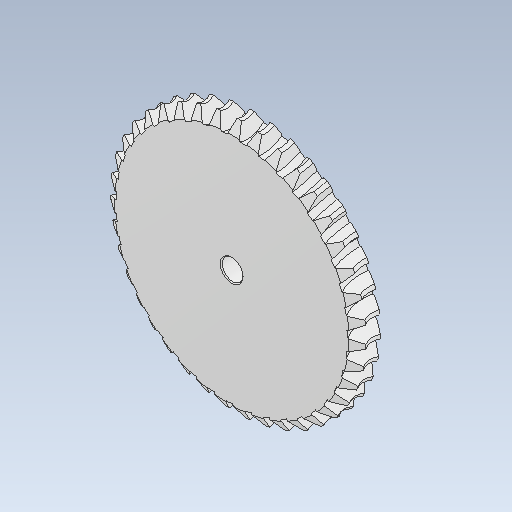
# Autodesk Inventor part: Worm Gear
Saved by Autodesk Inventor 2020 (Build 240168000, 168)
## iProperties
CustomPartVersion: 1
Created: 2020-05-17
Part Number: Worm Gear
Material: Acetal Resin, White
Document SubType Name: Modeling
Designer: Hesekiel
Categories: <?xml version="1.0" encoding="UTF-16"?> <MemberInstance><Categories><FamilyTemplate><FamilyTemplateParameter ValueType="xs:double" Id="1" ObjectReferenceKey="da_z" ObjectType="kUserParameterObject"/><FamilyTemplateParameter ValueType="xs:double" Id="2" ObjectReferenceKey="da_b" ObjectType="kUserParameterObject"/><FamilyTemplateParameter ValueType="xs:double" Id="3" ObjectReferenceKey="da_beta" ObjectType="kUserParameterObject"/><FamilyTemplateParameter ValueType="xs:double" Id="4" ObjectReferenceKey="da_m" ObjectType="kUserParameterObject"/><FamilyTemplateParameter ValueType="xs:double" Id="5" ObjectReferenceKey="da_alpha" ObjectType="kUserParameterObject"/><FamilyTemplateParameter ValueType="xs:double" Id="6" ObjectReferenceKey="da_da" ObjectType="kUserParameterObject"/><FamilyTemplateParameter ValueType="xs:double" Id="7" ObjectReferenceKey="da_aw" ObjectType="kUserParameterObject"/><FamilyTemplateParameter ValueType="xs:double" Id="8" ObjectReferenceKey="da_px" ObjectType="kUserParameterObject"/><FamilyTemplateParameter ValueType="xs:double" Id="9" ObjectReferenceKey="da_d" ObjectType="kUserParameterObject"/><FamilyTemplateParameter ValueType="xs:double" Id="10" ObjectReferenceKey="da_dae" ObjectType="kUserParameterObject"/><FamilyTemplateParameter ValueType="xs:double" Id="11" ObjectReferenceKey="da_fi" ObjectType="kUserParameterObject"/><FamilyTemplateParameter ValueType="xs:string" Id="12" ObjectReferenceKey="EAIAABAAAAAWFwAAAAAAAIAAAAAAAAAA" ObjectType="83910656" SubObjectId="SurfaceGeometry"/></FamilyTemplate><ParamToTemplateMap><ParamToTemplate CategoryParameter="//CategoryParameter[@InternalName='046C89C9-8512-4d59-83FE-43B91F4F132A']" TemplateParameter="1"/><ParamToTemplate CategoryParameter="//CategoryParameter[@InternalName='2552DF32-E462-4b46-AEBF-C6C7768E72AC']" TemplateParameter="2"/><ParamToTemplate CategoryParameter="//CategoryParameter[@InternalName='C9EE641D-15FC-4fae-A226-E94C4372FDD7']" TemplateParameter="3"/><ParamToTemplate><ParamToTemplate CategoryParameter="//CategoryParameter[@InternalName='00B6519A-459B-49c7-AD84-2E56D39A5744']" ConstantValue="-0.427778"/></ParamToTemplate><ParamToTemplate><ParamToTemplate CategoryParameter="//CategoryParameter[@InternalName='04B31F0E-C7A6-4894-AA32-9629BEFACF47']" ConstantValue="1.000000"/></ParamToTemplate><ParamToTemplate><ParamToTemplate CategoryParameter="//CategoryParameter[@InternalName='43CBEC2E-7847-49e7-A936-2F7889FCB2D9']" ConstantValue="0.200000"/></ParamToTemplate><ParamToTemplate><ParamToTemplate CategoryParameter="//CategoryParameter[@InternalName='B1EFC894-105D-4ebd-86BF-FA20ED196853']" ConstantValue="0.300000"/></ParamToTemplate><ParamToTemplate><ParamToTemplate CategoryParameter="//CategoryParameter[@InternalName='51175063-3D10-4879-93E8-6246FE8B403D']" ConstantValue="2060000000.000000"/></ParamToTemplate><ParamToTemplate><ParamToTemplate CategoryParameter="//CategoryParameter[@InternalName='A3A52E27-4454-46a9-B0BD-C932399B70AF']" ConstantValue="0.300000"/></ParamToTemplate><ParamToTemplate CategoryParameter="//CategoryParameter[@InternalName='91B76062-C214-41d9-B1B9-14D2AB99603D']" TemplateParameter="4"/><ParamToTemplate CategoryParameter="//CategoryParameter[@InternalName='2D373A89-B862-43d6-8D0B-0CBF12AB9F6C']" TemplateParameter="5"/><ParamToTemplate CategoryParameter="//CategoryParameter[@InternalName='37777632-D6A2-4fac-9D53-DB8ACD95C989']" TemplateParameter="6"/><ParamToTemplate CategoryParameter="//CategoryParameter[@InternalName='FD1017F1-B727-4f7e-9707-0F86F1FF9423']" TemplateParameter="7"/><ParamToTemplate CategoryParameter="//CategoryParameter[@InternalName='3BF567DA-17EF-48d8-80EA-D119B07F6463']" TemplateParameter="8"/><ParamToTemplate CategoryParameter="//CategoryParameter[@InternalName='BF5A1E7E-5373-4a22-AAD3-F583781FCF3C']" TemplateParameter="9"/><ParamToTemplate CategoryParameter="//CategoryParameter[@InternalName='2A200944-5A8C-41ca-B96E-8520D2E510F1']" TemplateParameter="10"/><ParamToTemplate CategoryParameter="//CategoryParameter[@InternalName='E77AC4FD-7B43-4566-B0ED-7CA70B976BC8']" TemplateParameter="11"/><ParamToTemplate><ParamToTemplate CategoryParameter="//CategoryParameter[@InternalName='D4F72237-D604-435a-AD0B-F738B7463A00']" ConstantValue="110.000000"/></ParamToTemplate><ParamToTemplate><ParamToTemplate CategoryParameter="//CategoryParameter[@InternalName='9E1B4470-B2D3-4ff1-B813-535BB4CDF51A']" ConstantValue="2000000.000000"/></ParamToTemplate><ParamToTemplate><ParamToTemplate CategoryParameter="//CategoryParameter[@InternalName='A7A89E9A-52E6-4d4f-86CF-A81914F22AA4']" ConstantValue="250000000.000000"/></ParamToTemplate><ParamToTemplate><ParamToTemplate CategoryParameter="//CategoryParameter[@InternalName='B02FABAC-469F-4ad8-A219-DB4578299DF6']" ConstantValue="250000000.000000"/></ParamToTemplate><ParamToTemplate><ParamToTemplate CategoryParameter="//CategoryParameter[@InternalName='E6981962-40D5-4343-A0AD-C263FCC47E10']" ConstantValue="9.000000"/></ParamToTemplate><ParamToTemplate><ParamToTemplate CategoryParameter="//CategoryParameter[@InternalName='B958E99F-2BCD-4955-8634-793EB7B37B89']" ConstantValue="8.000000"/></ParamToTemplate><ParamToTemplate><ParamToTemplate CategoryParameter="//CategoryParameter[@InternalName='4AD49A87-569D-440f-A541-E3B52A6A9DCE']" ConstantValue="1200.000000"/></ParamToTemplate><ParamToTemplate><ParamToTemplate CategoryParameter="//CategoryParameter[@InternalName='4E5813A0-330D-4b41-BE23-D880B01A1D55']" ConstantValue="1650000.000000"/></ParamToTemplate><ParamToTemplate><ParamToTemplate CategoryParameter="//CategoryParameter[@InternalName='19EB8C86-AA88-4253-B4AA-2F5DF1CE171A']" ConstantValue="6000.000000"/></ParamToTemplate><ParamToTemplate CategoryParameter="//CategoryParameter[@InternalName='27C3BAF2-7550-4e4b-AE2C-0DB134B7D9B7']" TemplateParameter="12"/></ParamToTemplateMap><Category DisplayName="Gear" InternalName="DC85795E-93AB-48d5-8EEE-5A27447B64BD" Mnemonic="Gear"><CategoryParameter DisplayName="z" InternalName="046C89C9-8512-4d59-83FE-43B91F4F132A" Mnemonic="z"/><CategoryParameter DisplayName="b|.2|" InternalName="2552DF32-E462-4b46-AEBF-C6C7768E72AC" Mnemonic="b"/><CategoryParameter DisplayName="||b|" InternalName="C9EE641D-15FC-4fae-A226-E94C4372FDD7" Mnemonic="beta"/><CategoryParameter DisplayName="x" InternalName="00B6519A-459B-49c7-AD84-2E56D39A5744" Mnemonic="x"/><CategoryParameter DisplayName="a*" InternalName="04B31F0E-C7A6-4894-AA32-9629BEFACF47" Mnemonic="a"/><CategoryParameter DisplayName="c*" InternalName="43CBEC2E-7847-49e7-A936-2F7889FCB2D9" Mnemonic="c"/><CategoryParameter DisplayName="r|.f|*" InternalName="B1EFC894-105D-4ebd-86BF-FA20ED196853" Mnemonic="rf"/><CategoryParameter DisplayName="E" InternalName="51175063-3D10-4879-93E8-6246FE8B403D" Mnemonic="E"/><CategoryParameter DisplayName="||m|" InternalName="A3A52E27-4454-46a9-B0BD-C932399B70AF" Mnemonic="mi"/><Category DisplayName="WormGear" InternalName="1B25C7EF-093B-4025-B3D3-619CD2A4550C" Mnemonic="WormGear"><CategoryParameter DisplayName="m" InternalName="91B76062-C214-41d9-B1B9-14D2AB99603D" Mnemonic="m"/><CategoryParameter DisplayName="||a|" InternalName="2D373A89-B862-43d6-8D0B-0CBF12AB9F6C" Mnemonic="alpha"/><CategoryParameter DisplayName="d|.a|" InternalName="37777632-D6A2-4fac-9D53-DB8ACD95C989" Mnemonic="da"/><CategoryParameter DisplayName="a|.w|" InternalName="FD1017F1-B727-4f7e-9707-0F86F1FF9423" Mnemonic="aw"/><CategoryParameter DisplayName="p|.x|" InternalName="3BF567DA-17EF-48d8-80EA-D119B07F6463" Mnemonic="px"/><CategoryParameter DisplayName="d" InternalName="BF5A1E7E-5373-4a22-AAD3-F583781FCF3C" Mnemonic="d"/><CategoryParameter DisplayName="dae" InternalName="2A200944-5A8C-41ca-B96E-8520D2E510F1" Mnemonic="dae"/><CategoryParameter DisplayName="||d|" InternalName="E77AC4FD-7B43-4566-B0ED-7CA70B976BC8" Mnemonic="fi"/><CategoryParameter DisplayName="VHV" InternalName="D4F72237-D604-435a-AD0B-F738B7463A00" Mnemonic="VHV"/><CategoryParameter DisplayName="||s||.Hlim|" InternalName="9E1B4470-B2D3-4ff1-B813-535BB4CDF51A" Mnemonic="sHlim"/><CategoryParameter DisplayName="N|.Flim|" InternalName="A7A89E9A-52E6-4d4f-86CF-A81914F22AA4" Mnemonic="NFlim"/><CategoryParameter DisplayName="N|.Hlim|" InternalName="B02FABAC-469F-4ad8-A219-DB4578299DF6" Mnemonic="NHlim"/><CategoryParameter DisplayName="q|.F|" InternalName="E6981962-40D5-4343-A0AD-C263FCC47E10" Mnemonic="qF"/><CategoryParameter DisplayName="q|.H|" InternalName="B958E99F-2BCD-4955-8634-793EB7B37B89" Mnemonic="qH"/><CategoryParameter DisplayName="v|.max|" InternalName="4AD49A87-569D-440f-A541-E3B52A6A9DCE" Mnemonic="maxv"/><CategoryParameter DisplayName="S|.n|" InternalName="4E5813A0-330D-4b41-BE23-D880B01A1D55" Mnemonic="Sn"/><CategoryParameter DisplayName="K|.w|" InternalName="19EB8C86-AA88-4253-B4AA-2F5DF1CE171A" Mnemonic="Kw"/><CategoryParameter DisplayName="PitchDiameter" InternalName="27C3BAF2-7550-4e4b-AE2C-0DB134B7D9B7" Mnemonic="IDS_PITCHDIAM"/></Category></Category></Categories></MemberInstance>
Density: 1.425 g/cm^3
Appearance: Smooth - White
Mass: 648.268 g
Surface Area: 690.453 cm^2
Volume: 454.925 cm^3
Author: Hesekiel
Autodesk Inventor part; units mm, degrees
ref_plane "Tooth Plane" through (0, -10, 0) normal (-0.1567675, 0, 0.9876355) x (0, 1, 0)
sketch "Base Body Sketch" plane through (0, 0, 0) normal (1, 0, 0) x (0, 1, 0)
  line L0 (0, -14) -> (0, 14) projected
  line L1 (0, 10) -> (84.228, 10)
  line L2 (84.228, 10) -> (92.575, 4.7077)
  line L3 (-21.935, 0) -> (131.61, 0) construction
  circle A0 centre (100, 0) radius 9.675
  line L4 (92.575, 4.7077) -> (92.575, -4.7077)
  line L5 (0, -10) -> (84.228, -10)
  line L6 (0, 10) -> (0, -10)
  line L7 (84.228, -10) -> (92.575, -4.7077)
  dimension "d50" = 32.376
  dimension "d87" = 185.15
  dimension "d89" = 19.35
  dimension "d92" = 20
  dimension "d93" = 100
  constraints: 14 end point, 3 symmetric about line, 2 perpendicular, 2 point on line, 1 centre point, 1 collinear
  measures "d50" angle of L2 L1
  measures "d87" diameter of L4 L0
  measures "d89" diameter of A0
  measures "d92" distance of L1.start L5.start
  measures "d93" distance from line of A0.centre L6
revolve "Base Body" add sketch "Base Body Sketch" angle 360 about axis through (0, 0, 0) along (0, 0, 1) picked at (91.8456, 0.3637) contours L0 L1 L2 A0 L7 L5 | A0 L2 L4 L7
revolve "Base Body2" cut sketch "Base Body Sketch" angle 360 about axis through (0, 0, 0) along (0, 0, 1) contours L7 L4 L2 A0 | A0 L2 L4 L7
sketch "Tooth Sketch" plane through (0, -10, 0) normal (-0.1567675, 0, 0.9876355) x (0, 1, 0)
  line L0 (10, 8.6892) -> (10, -8.6892) projected
  line L1 (-93.915, 0) -> (-66.51, 0) projected
  line L2 (-90, 6.2066) -> (-90, -6.2066)
  line L3 (-90, -6.2066) -> (-81.225, -6.2066)
  line L4 (-81.225, -6.2066) -> (-70.425, -2.2757)
  line L5 (-70.425, -2.2757) -> (-70.425, 0)
  line L6 (-70.425, 2.2757) -> (-81.225, 6.2066)
  line L7 (-81.225, 6.2066) -> (-90, 6.2066)
  line L8 (-70.425, 2.2757) -> (-70.425, 0)
  line L9 (-75.825, 0) -> (-75.825, -4.2412) construction
  dimension "d38" = 100
  dimension "d39" = 20
  dimension "d40" = 8.775
  dimension "d41" = 14.175
  dimension "d42" = 4.2412
  constraints: 16 end point, 4 perpendicular, 3 equal length, 2 point on line, 1 midpoint, 1 parallel, 1 vertical
  measures "d38" distance between parallel lines of L0 L2
  measures "d39" angle of L6 L7
  measures "d40" distance of L6.end L2.start
  measures "d41" distance between parallel lines of L2 L9
  measures "d42" distance of L9.start L9.end
sketch "Sketch8" plane through (0, 0, 10) normal (0, 0, 1) x (1, 0, 0)
  circle A0 centre (0, 0) radius 84.228 projected
  circle A1 centre (0, 0) radius 87.75
  dimension "d77" = 175.5
  constraints: 1 centre point, 1 coincident
  measures "d77" diameter of A1
surface extrude "Pitch Diameter" sketch "Sketch8" against normal blind 20 shown no curves A1
ref_plane "Work Plane13" through (0, 0, 0) normal (-0.0804666, 0.9967573, 0) x (0, 0, 1)
revolve "Tooth" cut sketch "Tooth Sketch" angle 360 about axis through (-6.1298, -100, -0.973) along (0.9876355, 0, 0.1567675)
pattern_circular "Tooth Pattern" count 39 over 360 about axis through (0, 0, 0) along (0, 0, 1) of "Tooth"
ref_plane "Work Plane14" through (0, 0, 0) normal (0.9967573, 0.0804666, 0) x (0, 0, 1)
ref_plane "Work Plane15" through (0, 0, 0) normal (0, -1, 0) x (0, 0, 1)
ref_plane "Work Plane17" through (0, 0, -10) normal (0, 0, 1) x (1, 0, 0)
ref_plane "Work Plane16" through (0, 12.5, -10) normal (0, 1, 0) x (-1, 0, 0)
sketch "Sketch14" plane through (0, 0, 10) normal (0, 0, 1) x (0.9951744, -0.0981218, 0)
  circle A0 centre (0, 0) radius 12.5
  circle A1 centre (0, 0) radius 7.5
  dimension "d109" = 25
  dimension "d110" = 15
  constraints: 2 centre point, 2 coincident
  measures "d109" diameter of A0
  measures "d110" diameter of A1
extrude "Extrusion6" [suppressed]
ref_plane "Work Plane18" through (0, 12.5, 10) normal (0, 1, 0) x (-1, 0, 0)
sketch "Sketch15" plane through (0, 12.5, 10) normal (0, 1, 0) x (-1, 0, 0)
  line L0 (12.5, 15) -> (-12.5, 15) projected
  line L1 (-12.5, 0) -> (12.5, 0) projected
  line L2 (0, 15) -> (0, 0)
  line L3 (7.5, 0) -> (-7.5, 0) projected
  circle A0 centre (0, 7.5) radius 3
  point P0 (0, -10)
  dimension "d113" = 6
  constraints: 3 midpoint, 2 end point, 1 centre point
  measures "d113" diameter of A0
extrude "Extrusion7" [suppressed]
thread "Thread2" size "M6x0.75" class "6H" standard "ANSI Metric M Profile" full length
chamfer "Chamfer1" [suppressed]
sketch "Sketch17" plane through (0, 0, -10) normal (0, 0, -1) x (-0.9750312, 0.2220678, 0)
  circle A0 centre (0, 0) radius 12.5
  dimension "d123" = 25
  constraints: 1 centre point, 1 coincident
  measures "d123" diameter of A0
extrude "Extrusion9" add sketch "Sketch17" along normal blind 15
sketch "Sketch16" plane through (0, 0, 10) normal (0, 0, 1) x (1, 0, 0)
  circle A0 centre (0, 0) radius 7.5 projected
extrude "Extrusion8" [suppressed]
sketch "Sketch18" plane through (0, 0, -25) normal (0, 0, -1) x (-1, 0, 0)
  circle A0 centre (0, 0) radius 7.5
  dimension "d126" = 15
  constraints: 1 centre point, 1 coincident
  measures "d126" diameter of A0
extrude "Extrusion10" cut sketch "Sketch18" against normal up to surface (35 mm away)
ref_plane "Work Plane19" through (0, 12.5, -10) normal (0, 1, 0) x (-1, 0, 0)
sketch "Sketch19" plane through (0, 12.5, -10) normal (0, 1, 0) x (-1, 0, 0)
  line L0 (-12.5, -15) -> (12.5, -15) projected
  line L1 (12.5, 0) -> (-12.5, 0) projected
  line L2 (7.5, -15) -> (-7.5, -15) projected
  line L3 (0, -15) -> (0, 0)
  line L4 (12.5, 0) -> (-12.5, 0) projected
  circle A0 centre (0, -7.5) radius 3
  point P0 (0, 10)
  dimension "d129" = 6
  constraints: 3 midpoint, 2 end point, 1 centre point
  measures "d129" diameter of A0
extrude "Extrusion11" cut sketch "Sketch19" against normal up to surface round surface about axis through (0, 0, -25) along (0, 0, 1) radius 7.5 far side no
thread "Thread3" size "M6x0.75" class "6H" standard "ANSI Metric M Profile" full length
chamfer "Chamfer2" distance 0.7 angle 45 3 edges at (12.1879, -2.7758, -25) (7.5, 0, -25) (7.5, 0, 10)
equation "\"d50\" = da_fi"
equation "\"d87\" = da_dae"
equation "\"d89\" = 2 * da_aw - da_da"
equation "\"d92\" = da_b"
equation "\"d93\" = da_aw"
equation "\"d38\" = da_aw"
equation "\"d39\" = da_alfat"
equation "\"d40\" = 0.5 * da_df1"
equation "\"d41\" = 0.5 * da_d1"
equation "\"d42\" = 0.3 * da_px"
equation "\"d77\" = da_dw"
equation "\"d78\" = da_b"
equation "\"da_aw\" = 100"
equation "\"da_fi\" = 32.3761deg"
equation "\"da_b\" = 20"
equation "\"da_df\" = 160.85"
equation "\"da_da\" = 180.65"
equation "\"da_beta\" = 9.019322deg"
equation "\"da_alfat\" = 20deg"
equation "\"da_df1\" = 17.55"
equation "\"da_da1\" = 37.35"
equation "\"da_d1\" = 28.35"
equation "\"da_px\" = 14.137167"
equation "\"da_dw\" = 175.5"
equation "\"da_rightdir\" = 0"
equation "\"da_dae\" = 185.15"
body "Solid1"
body "Srf1"
